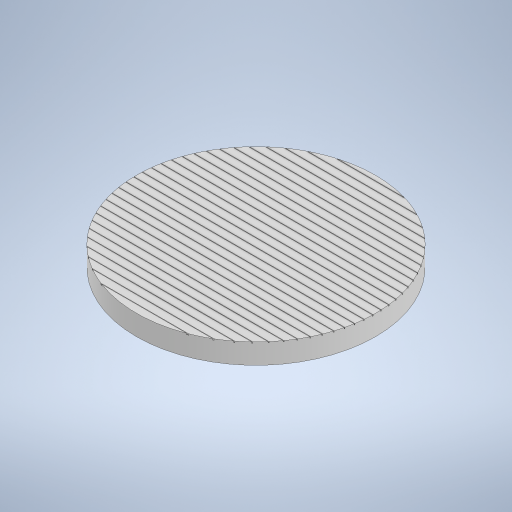
# Autodesk Inventor part: CircularTeflonHolder
Saved by Autodesk Inventor 2023 (Build 270158000, 158)
## iProperties
Created: 2023-08-11
Part Number: CircularTeflonHolder
Material: Generic
Document SubType Name: Modeling
Designer: Edwin
Density: 1 g/cm^3
Appearance: Default
Author: Edwin
Autodesk Inventor part; units mm, degrees
ref_plane "YZ Plane" through (0, 0, 0) normal (1, 0, 0) x (0, 1, 0)
ref_plane "XZ Plane" through (0, 0, 0) normal (0, 1, 0) x (-1, 0, 0)
ref_plane "XY Plane" through (0, 0, 0) normal (0, 0, 1) x (1, 0, 0)
sketch "Sketch1" plane through (0, 0, 0) normal (0, 1, 0) x (-1, 0, 0)
  circle A0 centre (0, 0) radius 100
  dimension "d0" = 200
  constraints: 1 centre point, 1 coincident
  measures "d0" diameter of A0
extrude "Extrusion1" add sketch "Sketch1" along normal blind 15
sketch "Sketch2" plane through (0, 0, 0) normal (0, -1, 0) x (1, 0, 0)
  circle A0 centre (0, 0) radius 100 projected
  circle A1 centre (0, 0) radius 80
  dimension "d3" = 20
  constraints: 1 centre point, 1 coincident
  measures "d3" radial gap between concentric circles of A0 A1
extrude "Extrusion2" add sketch "Sketch2" along normal blind 2
sketch "Sketch3" plane through (0, 0, 0) normal (1, 0, 0) x (0, 1, 0)
  line L0 (15, -100) -> (15, 100) projected
  line L1 (15, 100) -> (14, 100)
  line L2 (14, 100) -> (14, 100.5)
  line L3 (14, 100.5) -> (15, 100.5)
  line L4 (15, 100.5) -> (15, 100)
  line L5 (15, 93) -> (14, 93)
  line L6 (14, 93) -> (14, 93.5)
  line L7 (14, 93.5) -> (15, 93.5)
  line L8 (15, 93.5) -> (15, 93)
  line L9 (15, 86) -> (14, 86)
  line L10 (14, 86) -> (14, 86.5)
  line L11 (14, 86.5) -> (15, 86.5)
  line L12 (15, 86.5) -> (15, 86)
  line L13 (15, 79) -> (14, 79)
  line L14 (14, 79) -> (14, 79.5)
  line L15 (14, 79.5) -> (15, 79.5)
  line L16 (15, 79.5) -> (15, 79)
  line L17 (15, 72) -> (14, 72)
  line L18 (14, 72) -> (14, 72.5)
  line L19 (14, 72.5) -> (15, 72.5)
  line L20 (15, 72.5) -> (15, 72)
  line L21 (15, 65) -> (14, 65)
  line L22 (14, 65) -> (14, 65.5)
  line L23 (14, 65.5) -> (15, 65.5)
  line L24 (15, 65.5) -> (15, 65)
  line L25 (15, 58) -> (14, 58)
  line L26 (14, 58) -> (14, 58.5)
  line L27 (14, 58.5) -> (15, 58.5)
  line L28 (15, 58.5) -> (15, 58)
  line L29 (15, 51) -> (14, 51)
  line L30 (14, 51) -> (14, 51.5)
  line L31 (14, 51.5) -> (15, 51.5)
  line L32 (15, 51.5) -> (15, 51)
  line L33 (15, 44) -> (14, 44)
  line L34 (14, 44) -> (14, 44.5)
  line L35 (14, 44.5) -> (15, 44.5)
  line L36 (15, 44.5) -> (15, 44)
  line L37 (15, 37) -> (14, 37)
  line L38 (14, 37) -> (14, 37.5)
  line L39 (14, 37.5) -> (15, 37.5)
  line L40 (15, 37.5) -> (15, 37)
  line L41 (15, 30) -> (14, 30)
  line L42 (14, 30) -> (14, 30.5)
  line L43 (14, 30.5) -> (15, 30.5)
  line L44 (15, 30.5) -> (15, 30)
  line L45 (15, 23) -> (14, 23)
  line L46 (14, 23) -> (14, 23.5)
  line L47 (14, 23.5) -> (15, 23.5)
  line L48 (15, 23.5) -> (15, 23)
  line L49 (15, 16) -> (14, 16)
  line L50 (14, 16) -> (14, 16.5)
  line L51 (14, 16.5) -> (15, 16.5)
  line L52 (15, 16.5) -> (15, 16)
  line L53 (15, 9) -> (14, 9)
  line L54 (14, 9) -> (14, 9.5)
  line L55 (14, 9.5) -> (15, 9.5)
  line L56 (15, 9.5) -> (15, 9)
  line L57 (15, 2) -> (14, 2)
  line L58 (14, 2) -> (14, 2.5)
  line L59 (14, 2.5) -> (15, 2.5)
  line L60 (15, 2.5) -> (15, 2)
  line L61 (15, -5) -> (14, -5)
  line L62 (14, -5) -> (14, -4.5)
  line L63 (14, -4.5) -> (15, -4.5)
  line L64 (15, -4.5) -> (15, -5)
  line L65 (15, -12) -> (14, -12)
  line L66 (14, -12) -> (14, -11.5)
  line L67 (14, -11.5) -> (15, -11.5)
  line L68 (15, -11.5) -> (15, -12)
  line L69 (15, -19) -> (14, -19)
  line L70 (14, -19) -> (14, -18.5)
  line L71 (14, -18.5) -> (15, -18.5)
  line L72 (15, -18.5) -> (15, -19)
  line L73 (15, -26) -> (14, -26)
  line L74 (14, -26) -> (14, -25.5)
  line L75 (14, -25.5) -> (15, -25.5)
  line L76 (15, -25.5) -> (15, -26)
  line L77 (15, -33) -> (14, -33)
  line L78 (14, -33) -> (14, -32.5)
  line L79 (14, -32.5) -> (15, -32.5)
  line L80 (15, -32.5) -> (15, -33)
  line L81 (15, -40) -> (14, -40)
  line L82 (14, -40) -> (14, -39.5)
  line L83 (14, -39.5) -> (15, -39.5)
  line L84 (15, -39.5) -> (15, -40)
  line L85 (15, -47) -> (14, -47)
  line L86 (14, -47) -> (14, -46.5)
  line L87 (14, -46.5) -> (15, -46.5)
  line L88 (15, -46.5) -> (15, -47)
  line L89 (15, -54) -> (14, -54)
  line L90 (14, -54) -> (14, -53.5)
  line L91 (14, -53.5) -> (15, -53.5)
  line L92 (15, -53.5) -> (15, -54)
  line L93 (15, -61) -> (14, -61)
  line L94 (14, -61) -> (14, -60.5)
  line L95 (14, -60.5) -> (15, -60.5)
  line L96 (15, -60.5) -> (15, -61)
  line L97 (15, -68) -> (14, -68)
  line L98 (14, -68) -> (14, -67.5)
  line L99 (14, -67.5) -> (15, -67.5)
  line L100 (15, -67.5) -> (15, -68)
  line L101 (15, -75) -> (14, -75)
  line L102 (14, -75) -> (14, -74.5)
  line L103 (14, -74.5) -> (15, -74.5)
  line L104 (15, -74.5) -> (15, -75)
  line L105 (15, -82) -> (14, -82)
  line L106 (14, -82) -> (14, -81.5)
  line L107 (14, -81.5) -> (15, -81.5)
  line L108 (15, -81.5) -> (15, -82)
  line L109 (15, -89) -> (14, -89)
  line L110 (14, -89) -> (14, -88.5)
  line L111 (14, -88.5) -> (15, -88.5)
  line L112 (15, -88.5) -> (15, -89)
  line L113 (15, -96) -> (14, -96)
  line L114 (14, -96) -> (14, -95.5)
  line L115 (14, -95.5) -> (15, -95.5)
  line L116 (15, -95.5) -> (15, -96)
  point P0 (0, 0)
  dimension "d6" = 1
  dimension "d7" = 0.5
  dimension "d10" = 7
  constraints: 232 end point, 112 vertical alignment, 58 parallel, 56 collinear, 1 horizontal, 1 perpendicular, 1 other
  measures "d6" distance of L2.end L3.end
  measures "d7" distance of L1.end L2.end
  measures "d10" distance of L2.end L6.end
extrude "Extrusion3" cut sketch "Sketch3" along normal mid plane 200
body "Solid1"
